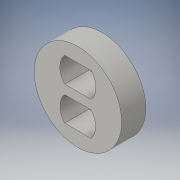
# Autodesk Inventor part: Zoetrope_Motor_Connector v2
Saved by Autodesk Inventor 2016 (Build 200138000, 138)
## iProperties
Created: 2019-01-08
Part Number: Zoetrope_Motor_Connector v2
Material: Generic
Document SubType Name: Modeling
Designer: student
Density: 1 g/cm^3
Appearance: Default
Author: student
Autodesk Inventor part; units mm, degrees
ref_plane "YZ Plane" through (0, 0, 0) normal (1, 0, 0) x (0, 1, 0)
ref_plane "XZ Plane" through (0, 0, 0) normal (0, 1, 0) x (-1, 0, 0)
ref_plane "XY Plane" through (0, 0, 0) normal (0, 0, 1) x (1, 0, 0)
sketch "Sketch1" plane through (0, 0, 0) normal (0, 0, 1) x (1, 0, 0)
  line L0 (0, 0) -> (5.0292, 0)
  line L1 (0, -4.7244) -> (5.0292, -4.7244)
  arc A0 (0, 0) -> (0, -4.7244) centre (2.594, -2.3622) ccw
  arc A1 (5.0292, -4.7244) -> (5.0292, 0) centre (2.4352, -2.3622) ccw
  line L2 (0, -6.438) -> (4.9784, -6.438)
  line L3 (0, -11.1116) -> (4.9784, -11.1116)
  arc A2 (0, -6.438) -> (0, -11.1116) centre (2.6267, -8.7748) ccw
  arc A3 (4.9784, -11.1116) -> (4.9784, -6.438) centre (2.3517, -8.7748) ccw
  circle A4 centre (2.5146, -5.5739) radius 8.2804
  dimension "d0" = 5.0292
  dimension "d2" = 5.0292
  dimension "d3" = 4.7244
  dimension "d8" = 3.5084
  dimension "d9" = 3.5084
  dimension "d10" = 0.1588
  dimension "d11" = 4.9784
  dimension "d12" = 4.6736
  dimension "d15" = 4.9784
  dimension "d16" = 3.5157
  dimension "d17" = 3.5157
  dimension "d18" = 6.7564
  constraints: 8 end point, 8 point on circle, 5 centre point, 4 horizontal
  measures "d0" distance of L0.start L0.end
  measures "d2" distance of L1.start L1.end
  measures "d3" distance between parallel lines of L1 L0
  measures "d8" radius of A0
  measures "d9" radius of A1
  measures "d10" distance of A0.centre A1.centre
  measures "d11" distance of L2.start L2.end
  measures "d12" distance between parallel lines of L3 L2
  measures "d15" distance of L3.start L3.end
  measures "d16" radius of A2
  measures "d17" radius of A3
extrude "Extrusion1" add sketch "Sketch1" along normal blind 4.572
body "Solid1"
